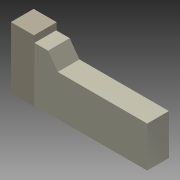
# Autodesk Inventor part: Selenoid Part 1764
Saved by Autodesk Inventor 2011 (Build 150239000, 239)
## iProperties
Created: 2010-02-15
Part Number: Selenoid Part 1764
Document SubType Name: Modeling
Designer: jgehrig
Density: 1 g/cm^3
Author: jgehrig
Autodesk Inventor part; units mm, degrees
ref_plane "YZ Plane" through (0, 0, 0) normal (1, 0, 0) x (0, 1, 0)
ref_plane "XZ Plane" through (0, 0, 0) normal (0, 1, 0) x (-1, 0, 0)
ref_plane "XY Plane" through (0, 0, 0) normal (0, 0, 1) x (1, 0, 0)
sketch "Sketch1" plane through (0, 0, 0) normal (0, 0, 1) x (1, 0, 0)
  line L0 (-36.6197, 6.2354) -> (-25.8247, 6.2354)
  line L1 (-25.8247, 6.2354) -> (-25.8247, -22.3396)
  line L2 (-25.8247, -22.3396) -> (-36.6197, -22.3396)
  line L3 (-36.6197, -22.3396) -> (-36.6197, 6.2354)
  line L4 (-25.8247, 3.0604) -> (-19.4747, 3.0604)
  line L5 (-19.4747, 3.0604) -> (-14.9147, -3.2896)
  line L6 (-14.9147, -3.2896) -> (26.9953, -3.2896)
  line L7 (26.9953, -3.2896) -> (26.9953, -22.3396)
  line L8 (26.9953, -22.3396) -> (-25.8247, -22.3396)
  point P0 (0, 0)
  dimension "d0" = 28.575
  dimension "d1" = 10.795
  dimension "d2" = 25.4
  dimension "d3" = 19.05
  dimension "d4" = 41.91
  dimension "d5" = 6.35
  constraints: 18 end point, 4 parallel, 3 perpendicular, 1 horizontal, 1 point on line
  measures "d0" distance of L2.end L0.start
  measures "d1" distance of L0.start L0.end
  measures "d2" distance between parallel lines of L8 L4
  measures "d3" distance of L6.end L7.end
  measures "d4" distance of L5.end L6.end
  measures "d5" distance of L4.start L4.end
extrude "Extrusion1" add sketch "Sketch1" along normal blind 10.16
sketch "Sketch2" plane through (0, 0, 0) normal (0, 0, -1) x (-1, 0, 0)
  line L0 (36.6197, -22.3396) -> (-26.9953, -22.3396) projected
  line L1 (36.6197, 6.2354) -> (25.8247, 6.2354)
  line L2 (25.8247, 6.2354) -> (25.8247, -22.3396)
  line L3 (25.8247, -22.3396) -> (36.6197, -22.3396)
  line L4 (36.6197, -22.3396) -> (36.6197, 6.2354)
  point P0 (0, 0)
  constraints: 8 end point, 2 parallel, 1 horizontal, 1 perpendicular, 1 point on line
extrude "Extrusion2" add sketch "Sketch2" along normal blind 0.254
sketch "Sketch3" plane through (0, 0, 10.16) normal (0, 0, 1) x (1, 0, 0)
  line L0 (26.9953, -22.3396) -> (-36.6197, -22.3396) projected
  line L1 (-36.6197, 6.2354) -> (-25.8247, 6.2354)
  line L2 (-25.8247, 6.2354) -> (-25.8247, -22.3396)
  line L3 (-25.8247, -22.3396) -> (-36.6197, -22.3396)
  line L4 (-36.6197, -22.3396) -> (-36.6197, 6.2354)
  point P0 (0, 0)
  constraints: 8 end point, 2 parallel, 1 horizontal, 1 perpendicular, 1 point on line
extrude "Extrusion3" add sketch "Sketch3" along normal blind 0.254
sketch "Sketch4" plane through (-25.8247, -22.3396, 0) normal (0, -1, 0) x (1, 0, 0)
  line L0 (-10.795, 10.414) -> (0, 10.414)
  line L1 (0, 10.414) -> (0, -0.254)
  line L2 (0, -0.254) -> (-10.795, -0.254)
  line L3 (-10.795, -0.254) -> (-10.795, 10.414)
  point P0 (25.8247, 0)
  constraints: 8 end point, 2 parallel, 1 horizontal, 1 perpendicular
extrude "Extrusion4" add sketch "Sketch4" along normal blind 0.254
body "Solid1"
